Autodesk Fusion 360 part; units mm, degrees
(part 4 of 6)
  spline S27 degree 5 poles (23.2819, -10.1545) (23.2739, -10.1416) (23.2579, -10.1158) (23.2338, -10.0772) (23.2015, -10.026) (23.1609, -9.9622) (23.12, -9.8988) (23.0788, -9.8357) (23.0374, -9.7729) (22.9956, -9.7104) (22.9537, -9.6483) (22.9114, -9.5865) (22.8688, -9.525) (22.826, -9.4639) (22.7829, -9.4031) (22.7396, -9.3426) (22.6959, -9.2826) (22.652, -9.2228) (22.6078, -9.1634) (22.5634, -9.1044) (22.5186, -9.0458) (22.4736, -8.9875) (22.4284, -8.9296) (22.3828, -8.872) (22.337, -8.8148) (22.2909, -8.7581) (22.2445, -8.7017) (22.1979, -8.6456) (22.151, -8.59) (22.1038, -8.5348) (22.0563, -8.48) (22.0086, -8.4256) (21.9606, -8.3716) (21.9123, -8.318) (21.8638, -8.2649) (21.8149, -8.2122) (21.7658, -8.1599) (21.7164, -8.108) (21.6668, -8.0566) (21.6168, -8.0056) (21.5666, -7.9551) (21.5161, -7.9051) (21.4653, -7.8556) (21.4143, -7.8065) (21.3629, -7.7579) (21.3113, -7.7099) (21.2594, -7.6623) (21.2072, -7.6152) (21.1547, -7.5686) (21.1019, -7.5225) (21.0489, -7.477) (20.9955, -7.4321) (20.9418, -7.3878) (20.8878, -7.3441) (20.8335, -7.3011) (20.7788, -7.2586) (20.7239, -7.2166) (20.6688, -7.1752) (20.6133, -7.1344) (20.5575, -7.0942) (20.5014, -7.0549) (20.4448, -7.0164) (20.3878, -6.979) (20.3303, -6.9426) (20.2724, -6.907) (20.2143, -6.8722) (20.1559, -6.8378) (20.0973, -6.8039) (20.0385, -6.7707) (19.9791, -6.7389) (19.919, -6.7091) (19.8699, -6.6876) (19.8324, -6.673) (19.8071, -6.6641) (19.7944, -6.6598) knots -1 -1 -1 -1 -1 -1 -0.98571429 -0.97142857 -0.95714286 -0.94285714 -0.92857143 -0.91428571 -0.9 -0.88571429 -0.87142857 -0.85714286 -0.84285714 -0.82857143 -0.81428571 -0.8 -0.78571429 -0.77142857 -0.75714286 -0.74285714 -0.72857143 -0.71428571 -0.7 -0.68571429 -0.67142857 -0.65714286 -0.64285714 -0.62857143 -0.61428571 -0.6 -0.58571429 -0.57142857 -0.55714286 -0.54285714 -0.52857143 -0.51428571 -0.5 -0.48571429 -0.47142857 -0.45714286 -0.44285714 -0.42857143 -0.41428571 -0.4 -0.38571429 -0.37142857 -0.35714286 -0.34285714 -0.32857143 -0.31428571 -0.3 -0.28571429 -0.27142857 -0.25714286 -0.24285714 -0.22857143 -0.21428571 -0.2 -0.18571429 -0.17142857 -0.15714286 -0.14285714 -0.12857143 -0.11428571 -0.1 -0.08571429 -0.07142857 -0.05714286 -0.04285714 -0.02857143 -0.01428571 0 0 0 0 0 0
  line L27 (19.7944, -6.6598) -> (18.8495, -6.3414)
  arc A59 (17.8163, -4.4521) -> (18.8495, -6.3414) centre (19.3565, -4.837) ccw
  line L28 (3.3592, 13.8919) -> (10.16, 13.8919)
  line L29 (10.16, 13.8919) -> (10.16, 101.6)
  line L30 (10.16, 101.6) -> (3.3592, 101.6)
  line L31 (3.3592, 35.7199) -> (-12.5468, 19.2505)
  line L32 (-10.3768, 14.5152) -> (3.3592, 18.3604)
  line L33 (-12.5468, 19.2505) -> (-10.3768, 14.5152)
  line L34 (3.3592, 101.6) -> (3.3592, 35.7199)
  line L35 (3.3592, 18.3604) -> (3.3592, 13.8919)
  line L36 (-55.9735, 14.1018) -> (-55.9735, 101.81)
  line L37 (-35.4367, 14.7251) -> (-49.1726, 18.5703)
  line L38 (-55.9735, 101.81) -> (-49.1726, 101.81)
  line L39 (-49.1726, 18.5703) -> (-49.1726, 14.1018)
  line L40 (-49.1726, 101.81) -> (-49.1726, 35.9298)
  line L41 (-49.1726, 35.9298) -> (-33.2667, 19.4605)
  line L42 (-33.2667, 19.4605) -> (-35.4367, 14.7251)
  line L43 (-49.1726, 14.1018) -> (-55.9735, 14.1018)
  constraint horizontal L28
  constraint vertical L29
  constraint horizontal L30
  constraint vertical L34
  constraint coincident S10 L31.end
  constraint coincident L32.end L34
  constraint collinear L34 L35
  constraint perpendicular L36 L43
extrude "Extrude3'" add sketch "Sketch3 (3)" against normal blind 12.7 contours A15 A16 A17 L6 S6 A18 S7 L7 A19 A20 A21 L8 S8 A22 S9 L9 A23 A24 A25 L10 S10 L29 L30 L31 L34 | L36 L37 L38 L39 L40 L41 L42 L43 sketch seen with x (0.965926, -0.258819, 0) y (0.258819, 0.965926, 0) z (0, 0, 1) at (44.1308, -10.9509, 0) bodies 2 makes body 3 at (65.5892, 29.8778, 8.4667) in component "Spur Gear (14 teeth) (1)"
sketch "Sketch4" plane through (3.3592, 0, 0) normal (-1, 0, 0) x (0, 0, 1)
  line L0 (12.7, 35.7199) -> (12.7, 101.6)
  line L1 (12.7, 101.6) -> (0, 101.6)
  line L2 (0, 101.6) -> (0, 35.7199)
  line L3 (0, 35.7199) -> (12.7, 35.7199)
  line L4 (12.7, 101.6) -> (23.6482, 101.6)
  line L5 (23.6482, 101.6) -> (23.6482, 52.5233)
  line L6 (12.9467, 36.0985) -> (12.7, 36.0985)
  line L7 (12.7, 36.0985) -> (12.7, 101.6)
  line L8 (12.7, 35.7199) -> (23.6482, 52.5233)
  constraint horizontal L4
  constraint vertical L5
  constraint horizontal L6
  constraint vertical L7
  constraint coincident L0.end L1.start
  constraint coincident L0.start L3.end
  constraint coincident L8 L6.start
extrude "Extrude4" add sketch "Sketch4" against normal blind 7.62 contours L0 L4 L5 L6 L7 L8 sketch seen with x (0.965926, -0.258819, 0) y (0.258819, 0.965926, 0) z (0, 0, 1) at (44.1308, -10.9509, 0) bodies 3 in component "Spur Gear (14 teeth) (1)"
ref_plane "WorkPlane1" through (-15.6908, 68.6599, 11.8241) normal (-1, 0, 0) x (0, 1, 0)
sketch "Sketch5" plane through (-15.6908, 0, 0) normal (-1, 0, 0) x (0, 0, 1)
  point P0 (12.6888, 89.7764)
sketch "Sketch6" plane through (3.3592, 0, 0) normal (-1, 0, 0) x (0, 0, 1)
  line L0 (23.6482, 101.6) -> (0, 101.6)
  line L1 (0, 101.6) -> (0, 35.7199)
  line L2 (0, 35.7199) -> (12.7, 35.7199)
  line L3 (12.7, 35.7199) -> (12.7, 36.0985)
  line L4 (12.7, 36.0985) -> (12.9467, 36.0985)
  line L5 (12.9467, 36.0985) -> (23.6482, 52.5233)
  line L6 (23.6482, 52.5233) -> (23.6482, 101.6)
  line L7 (0, 101.6) -> (23.6482, 101.6)
  line L8 (23.6482, 101.6) -> (23.6482, 77.0617)
  line L9 (23.6482, 77.0617) -> (0, 77.0617)
  line L10 (0, 77.0617) -> (0, 101.6)
  constraint horizontal L7
  constraint vertical L8
  constraint horizontal L9
  constraint vertical L10
  constraint midpoint L6 L8.end
  constraint coincident L0.end L1.start
loft "Loft1" add profiles "Sketch6" section 1 contours L0 L1 L6 L7 L8 L9 L10 sketch seen with x (0.965926, -0.258819, 0) y (0.258819, 0.965926, 0) z (0, 0, 1) at (44.1308, -10.9509, 0) section 2 point at (52.2104, 79.8275, 12.6888) bodies 3 in component "Spur Gear (14 teeth) (1)"
sketch "Sketch7" plane through (3.3592, 0, 0) normal (-1, 0, 0) x (0, 0, 1)
  line L0 (23.6482, 77.0617) -> (0, 77.0617)
  line L1 (0, 77.0617) -> (0, 35.7199)
  line L2 (0, 35.7199) -> (12.7, 35.7199)
  line L3 (12.7, 35.7199) -> (12.7, 36.0985)
  line L4 (12.7, 36.0985) -> (12.9467, 36.0985)
  line L5 (12.9467, 36.0985) -> (23.6482, 52.5233)
  line L6 (23.6482, 52.5233) -> (23.6482, 77.0617)
  line L7 (0, 77.0617) -> (23.6482, 77.0617)
  line L8 (23.6482, 77.0617) -> (23.6482, 55.8032)
  line L9 (23.6482, 55.8032) -> (0, 55.8032)
  line L10 (0, 55.8032) -> (0, 77.0617)
  constraint horizontal L7
  constraint vertical L8
  constraint horizontal L9
  constraint vertical L10
  constraint coincident L6 L8.end
  constraint coincident L0.end L1.start
ref_plane "WorkPlane2" through (-15.6908, 66.4325, 11.8241) normal (-1, 0, 0) x (0, 0, 1)
sketch "Sketch8" plane through (-15.6908, 0, 0) normal (-1, 0, 0) x (0, 0, 1)
  point P0 (12.5523, 67.1276)
loft "Loft2" add profiles "Sketch7" section 1 contours L0 L1 L6 L7 L8 L9 L10 sketch seen with x (0.965926, -0.258819, 0) y (0.258819, 0.965926, 0) z (0, 0, 1) at (44.1308, -10.9509, 0) section 2 point at (46.3485, 57.9505, 12.5523) bodies 3 in component "Spur Gear (14 teeth) (1)"
sketch "Sketch9" plane through (-49.1726, 0, 0) normal (1, 0, 0) x (0, 0, -1)
  line L0 (-12.7, 101.81) -> (-12.7, 35.9298)
  line L1 (-12.7, 35.9298) -> (0, 35.9298)
  line L2 (0, 35.9298) -> (0, 101.81)
  line L3 (0, 101.81) -> (-12.7, 101.81)
  line L4 (0, 101.81) -> (-23.6474, 101.81)
  line L5 (-23.6474, 101.81) -> (-23.6474, 52.5287)
  line L6 (0, 35.8833) -> (0, 101.81)
  line L7 (-12.7, 35.9298) -> (-23.6474, 52.5287)
  dimension "d33" = 23.6474
  constraint horizontal L4
  constraint vertical L5
  constraint vertical L6
  constraint coincident L2.end L3.start
  constraint coincident L0.end L1.start
  measures "d33" distance of L2.end L4.end
extrude "Extrude5" add sketch "Sketch9" against normal blind 6.731 contours L0 L4 L5 L7 sketch seen with x (0.965926, -0.258819, 0) y (0.258819, 0.965926, 0) z (0, 0, 1) at (44.1308, -10.9509, 0) bodies 2 in component "Spur Gear (14 teeth) (1)"
sketch "Sketch10" plane through (-49.1726, 0, 0) normal (1, 0, 0) x (0, 0, -1)
  line L0 (-12.7, 35.9298) -> (0, 35.9298)
  line L1 (0, 35.9298) -> (0, 101.81)
  line L2 (0, 101.81) -> (-23.6474, 101.81)
  line L3 (-23.6474, 101.81) -> (-23.6474, 52.5287)
  line L4 (-23.6474, 52.5287) -> (-12.7, 35.9298)
  line L5 (-23.6474, 101.81) -> (-0.1184, 101.81)
  line L6 (-0.1184, 101.81) -> (-0.1184, 77.2736)
  line L7 (-0.1184, 77.2736) -> (-23.6474, 77.2736)
  line L8 (-23.6474, 77.2736) -> (-23.6474, 101.81)
  line L9 (-23.6474, 77.2736) -> (0, 77.2736)
  line L10 (0, 77.2736) -> (0, 52.4632)
  line L11 (0, 52.4632) -> (-23.6474, 52.4632)
  line L12 (-23.6474, 52.4632) -> (-23.6474, 77.2736)
  dimension "d36" = 24.5364
  constraint horizontal L5
  constraint vertical L6
  constraint horizontal L7
  constraint vertical L8
  constraint coincident L2.end L3.start
  constraint horizontal L9
  constraint vertical L10
  constraint horizontal L11
  constraint vertical L12
  constraint coincident L1 L10.end
  measures "d36" distance of L2.end L7.end
ref_plane "WorkPlane3" through (-30.1226, 89.5418, 11.8829) normal (1, 0, 0) x (0, 0, -1)
ref_plane "WorkPlane4" through (-30.1226, 64.8684, 11.8237) normal (1, 0, 0) x (0, 0, -1)
sketch "Sketch11" plane through (-30.1226, 0, 0) normal (1, 0, 0) x (0, 0, -1)
  point P0 (-11.0515, 90.4417)
sketch "Sketch12" plane through (-49.1726, 0, 0) normal (1, 0, 0) x (0, 0, -1)
sketch "Sketch13" plane through (-30.1226, 0, 0) normal (1, 0, 0) x (0, 0, -1)
  point P0 (-11.1758, 64.0599)
loft "Loft3" add profiles "Sketch10" section 1 contours L2 L3 L5 L6 L7 L8 L9 sketch seen with x (0.965926, -0.258819, 0) y (0.258819, 0.965926, 0) z (0, 0, 1) at (44.1308, -10.9509, 0) section 2 point at (38.4426, 84.2054, 11.0515) bodies 2 in component "Spur Gear (14 teeth) (1)"
sketch "Sketch14" plane through (-49.1726, 0, 0) normal (1, 0, 0) x (0, 0, -1)
  line L0 (-0.1184, 101.81) -> (-0.1184, 77.2736)
  line L1 (-0.1184, 77.2736) -> (-23.6474, 77.2736)
  line L2 (-23.6474, 77.2736) -> (-23.6474, 52.5287)
  line L3 (-23.6474, 52.5287) -> (-12.7, 35.9298)
  line L4 (-12.7, 35.9298) -> (0, 35.9298)
  line L5 (0, 35.9298) -> (0, 101.81)
  line L6 (0, 101.81) -> (-0.1184, 101.81)
  line L7 (-23.6474, 77.2736) -> (0, 77.2736)
  line L8 (0, 77.2736) -> (0, 52.6508)
  line L9 (0, 52.6508) -> (-23.6474, 52.6508)
  line L10 (-23.6474, 52.6508) -> (-23.6474, 77.2736)
  constraint horizontal L7
  constraint vertical L8
  constraint horizontal L9
  constraint vertical L10
  constraint coincident L5 L8.end
  constraint coincident L1.end L2.start
loft "Loft4" add profiles "Sketch14" section 1 contours L1 L2 L5 L7 L8 L9 L10 sketch seen with x (0.965926, -0.258819, 0) y (0.258819, 0.965926, 0) z (0, 0, 1) at (44.1308, -10.9509, 0) section 2 point at (31.6145, 58.7226, 11.1758) bodies 2 in component "Spur Gear (14 teeth) (1)"
sketch "Sketch15" plane through (0, 0, 12.7) normal (0, 0, 1) x (1, 0, 0)
  line L0 (-55.9036, 35.9298) -> (-55.9036, 101.81)
  line L1 (-55.9036, 101.81) -> (-55.9735, 101.81)
  line L2 (-55.9735, 101.81) -> (-55.9735, 21.7403)
  spline S0 degree 5 poles (-55.9735, 21.7403) (-55.9837, 21.7467) (-56.0067, 21.761) (-56.0426, 21.7832) (-56.0913, 21.8132) (-56.1531, 21.8508) (-56.2177, 21.8896) (-56.2826, 21.928) (-56.3479, 21.9663) (-56.4003, 21.9966) (-56.4398, 22.0192) (-56.4661, 22.0343) (-56.4794, 22.0418) knots 0.888467 0.888467 0.888467 0.888467 0.888467 0.888467 0.9 0.914286 0.928571 0.942857 0.957143 0.971429 0.985714 1 1 1 1 1 1
  arc A0 (-56.4794, 22.0418) -> (-58.1639, 21.1514) centre (-45.4614, -0.8441) ccw
  spline S1 degree 5 poles (-58.1639, 21.1514) (-58.1652, 21.1363) (-58.1676, 21.106) (-58.1712, 21.0607) (-58.1756, 21.0003) (-58.1808, 20.9248) (-58.1856, 20.8495) (-58.1899, 20.7743) (-58.1939, 20.6991) (-58.1974, 20.6241) (-58.2005, 20.5492) (-58.2032, 20.4743) (-58.2055, 20.3996) (-58.2073, 20.325) (-58.2087, 20.2505) (-58.2097, 20.1761) (-58.2103, 20.1019) (-58.2104, 20.0277) (-58.2101, 19.9537) (-58.2094, 19.8798) (-58.2083, 19.8061) (-58.2067, 19.7325) (-58.2046, 19.659) (-58.2022, 19.5856) (-58.1992, 19.5124) (-58.1959, 19.4394) (-58.1921, 19.3665) (-58.1878, 19.2937) (-58.1831, 19.2211) (-58.1779, 19.1486) (-58.1723, 19.0763) (-58.1662, 19.0042) (-58.1596, 18.9323) (-58.1526, 18.8605) (-58.1451, 18.7889) (-58.1371, 18.7175) (-58.1286, 18.6463) (-58.1197, 18.5752) (-58.1102, 18.5044) (-58.1003, 18.4337) (-58.0899, 18.3632) (-58.079, 18.293) (-58.0675, 18.223) (-58.0556, 18.1532) (-58.0431, 18.0836) (-58.0301, 18.0143) (-58.0166, 17.9451) (-58.0026, 17.8763) (-57.988, 17.8076) (-57.9729, 17.7392) (-57.9572, 17.6711) (-57.941, 17.6033) (-57.9241, 17.5357) (-57.9065, 17.4685) (-57.8884, 17.4016) (-57.8697, 17.335) (-57.8504, 17.2686) (-57.8306, 17.2025) (-57.8103, 17.1368) (-57.7892, 17.0713) (-57.7674, 17.0063) (-57.7447, 16.9418) (-57.7211, 16.8778) (-57.6965, 16.8144) (-57.671, 16.7514) (-57.6449, 16.6888) (-57.6183, 16.6265) (-57.5913, 16.5645) (-57.5637, 16.5029) (-57.5349, 16.442) (-57.5041, 16.3822) (-57.4774, 16.3358) (-57.4559, 16.3018) (-57.4408, 16.2796) (-57.4332, 16.2686) knots -1 -1 -1 -1 -1 -1 -0.98571429 -0.97142857 -0.95714286 -0.94285714 -0.92857143 -0.91428571 -0.9 -0.88571429 -0.87142857 -0.85714286 -0.84285714 -0.82857143 -0.81428571 -0.8 -0.78571429 -0.77142857 -0.75714286 -0.74285714 -0.72857143 -0.71428571 -0.7 -0.68571429 -0.67142857 -0.65714286 -0.64285714 -0.62857143 -0.61428571 -0.6 -0.58571429 -0.57142857 -0.55714286 -0.54285714 -0.52857143 -0.51428571 -0.5 -0.48571429 -0.47142857 -0.45714286 -0.44285714 -0.42857143 -0.41428571 -0.4 -0.38571429 -0.37142857 -0.35714286 -0.34285714 -0.32857143 -0.31428571 -0.3 -0.28571429 -0.27142857 -0.25714286 -0.24285714 -0.22857143 -0.21428571 -0.2 -0.18571429 -0.17142857 -0.15714286 -0.14285714 -0.12857143 -0.11428571 -0.1 -0.08571429 -0.07142857 -0.05714286 -0.04285714 -0.02857143 -0.01428571 0 0 0 0 0 0
  line L3 (-57.4332, 16.2686) -> (-56.862, 15.4514)
  arc A1 (-57.1526, 13.3178) -> (-56.862, 15.4514) centre (-58.1632, 14.542) ccw
  arc A2 (-57.1526, 13.3178) -> (-57.7226, 12.8272) centre (-45.4614, -0.8441) ccw
  arc A3 (-59.8757, 12.8579) -> (-57.7226, 12.8272) centre (-58.7825, 14.009) ccw
  line L4 (-59.8757, 12.8579) -> (-60.5987, 13.5444)
  spline S2 degree 5 poles (-60.5987, 13.5444) (-60.6084, 13.5537) (-60.6281, 13.5719) (-60.6585, 13.5982) (-60.7005, 13.6316) (-60.7549, 13.6709) (-60.8109, 13.7084) (-60.8677, 13.745) (-60.925, 13.7809) (-60.9826, 13.8165) (-61.0407, 13.8516) (-61.0991, 13.8862) (-61.1582, 13.92) (-61.2179, 13.9529) (-61.2783, 13.9849) (-61.3394, 14.0162) (-61.401, 14.0467) (-61.463, 14.0767) (-61.5253, 14.1061) (-61.5881, 14.135) (-61.6512, 14.1635) (-61.7146, 14.1914) (-61.7785, 14.2187) (-61.8428, 14.2455) (-61.9074, 14.2717) (-61.9724, 14.2973) (-62.0378, 14.3225) (-62.1035, 14.3471) (-62.1695, 14.3712) (-62.2359, 14.3949) (-62.3025, 14.4181) (-62.3695, 14.4408) (-62.4367, 14.463) (-62.5042, 14.4848) (-62.5721, 14.506) (-62.6402, 14.5268) (-62.7086, 14.5472) (-62.7772, 14.5671) (-62.8461, 14.5865) (-62.9153, 14.6055) (-62.9847, 14.624) (-63.0544, 14.6421) (-63.1243, 14.6598) (-63.1945, 14.677) (-63.2649, 14.6938) (-63.3356, 14.7101) (-63.4064, 14.726) (-63.4775, 14.7415) (-63.5488, 14.7566) (-63.6204, 14.7712) (-63.6921, 14.7854) (-63.7641, 14.7992) (-63.8362, 14.8126) (-63.9086, 14.8256) (-63.9811, 14.8381) (-64.0539, 14.8503) (-64.1269, 14.862) (-64.2, 14.8733) (-64.2733, 14.8842) (-64.3468, 14.8947) (-64.4205, 14.9048) (-64.4944, 14.9145) (-64.5685, 14.9238) (-64.6427, 14.9327) (-64.7171, 14.9412) (-64.7916, 14.9493) (-64.8664, 14.957) (-64.9412, 14.9643) (-65.0163, 14.9712) (-65.0915, 14.9777) (-65.1668, 14.9838) (-65.2272, 14.9884) (-65.2726, 14.9917) (-65.3029, 14.9938) (-65.318, 14.9948) knots 0 0 0 0 0 0 0.01428571 0.02857143 0.04285714 0.05714286 0.07142857 0.08571429 0.1 0.11428571 0.12857143 0.14285714 0.15714286 0.17142857 0.18571429 0.2 0.21428571 0.22857143 0.24285714 0.25714286 0.27142857 0.28571429 0.3 0.31428571 0.32857143 0.34285714 0.35714286 0.37142857 0.38571429 0.4 0.41428571 0.42857143 0.44285714 0.45714286 0.47142857 0.48571429 0.5 0.51428571 0.52857143 0.54285714 0.55714286 0.57142857 0.58571429 0.6 0.61428571 0.62857143 0.64285714 0.65714286 0.67142857 0.68571429 0.7 0.71428571 0.72857143 0.74285714 0.75714286 0.77142857 0.78571429 0.8 0.81428571 0.82857143 0.84285714 0.85714286 0.87142857 0.88571429 0.9 0.91428571 0.92857143 0.94285714 0.95714286 0.97142857 0.98571429 1 1 1 1 1 1
  arc A4 (-65.318, 14.9948) -> (-66.4495, 13.4617) centre (-45.4614, -0.8441) ccw
  spline S3 degree 5 poles (-66.4495, 13.4617) (-66.4441, 13.4476) (-66.4331, 13.4192) (-66.4166, 13.3768) (-66.3945, 13.3205) (-66.3664, 13.2503) (-66.338, 13.1803) (-66.3093, 13.1107) (-66.2802, 13.0413) (-66.2509, 12.9721) (-66.2211, 12.9033) (-66.1911, 12.8347) (-66.1607, 12.7664) (-66.13, 12.6984) (-66.099, 12.6306) (-66.0676, 12.5632) (-66.0359, 12.496) (-66.0039, 12.4292) (-65.9715, 12.3626) (-65.9388, 12.2964) (-65.9057, 12.2304) (-65.8723, 12.1648) (-65.8386, 12.0994) (-65.8046, 12.0344) (-65.7702, 11.9697) (-65.7354, 11.9054) (-65.7004, 11.8413) (-65.665, 11.7776) (-65.6292, 11.7143) (-65.5931, 11.6512) (-65.5567, 11.5885) (-65.5199, 11.5262) (-65.4828, 11.4642) (-65.4453, 11.4026) (-65.4074, 11.3414) (-65.3693, 11.2805) (-65.3307, 11.22) (-65.2918, 11.1599) (-65.2526, 11.1001) (-65.213, 11.0408) (-65.1731, 10.9818) (-65.1327, 10.9233) (-65.0921, 10.8651) (-65.051, 10.8074) (-65.0096, 10.7502) (-64.9678, 10.6933) (-64.9256, 10.6369) (-64.8831, 10.5809) (-64.8402, 10.5254) (-64.7969, 10.4703) (-64.7532, 10.4158) (-64.7091, 10.3617) (-64.6646, 10.3082) (-64.6196, 10.2552) (-64.5743, 10.2028) (-64.5285, 10.1509) (-64.4824, 10.0995) (-64.4359, 10.0485) (-64.389, 9.9981) (-64.3416, 9.9483) (-64.2938, 9.8992) (-64.2453, 9.8509) (-64.1963, 9.8035) (-64.1466, 9.757) (-64.0963, 9.7113) (-64.0456, 9.6663) (-63.9947, 9.6217) (-63.9434, 9.5775) (-63.8918, 9.534) (-63.8394, 9.4916) (-63.7858, 9.4511) (-63.7415, 9.4209) (-63.7074, 9.3996) (-63.6842, 9.3861) (-63.6725, 9.3795) knots -1 -1 -1 -1 -1 -1 -0.98571429 -0.97142857 -0.95714286 -0.94285714 -0.92857143 -0.91428571 -0.9 -0.88571429 -0.87142857 -0.85714286 -0.84285714 -0.82857143 -0.81428571 -0.8 -0.78571429 -0.77142857 -0.75714286 -0.74285714 -0.72857143 -0.71428571 -0.7 -0.68571429 -0.67142857 -0.65714286 -0.64285714 -0.62857143 -0.61428571 -0.6 -0.58571429 -0.57142857 -0.55714286 -0.54285714 -0.52857143 -0.51428571 -0.5 -0.48571429 -0.47142857 -0.45714286 -0.44285714 -0.42857143 -0.41428571 -0.4 -0.38571429 -0.37142857 -0.35714286 -0.34285714 -0.32857143 -0.31428571 -0.3 -0.28571429 -0.27142857 -0.25714286 -0.24285714 -0.22857143 -0.21428571 -0.2 -0.18571429 -0.17142857 -0.15714286 -0.14285714 -0.12857143 -0.11428571 -0.1 -0.08571429 -0.07142857 -0.05714286 -0.04285714 -0.02857143 -0.01428571 0 0 0 0 0 0
  line L5 (-63.6725, 9.3795) -> (-62.8034, 8.891)
  arc A5 (-62.1394, 6.8427) -> (-62.8034, 8.891) centre (-63.5812, 7.5071) ccw
  arc A6 (-62.1394, 6.8427) -> (-62.4401, 6.1534) centre (-45.4614, -0.8441) ccw
  arc A7 (-64.3933, 5.2468) -> (-62.4401, 6.1534) centre (-63.9079, 6.7583) ccw
  line L6 (-64.3933, 5.2468) -> (-65.3426, 5.5517)
  spline S4 degree 5 poles (-65.3426, 5.5517) (-65.3554, 5.5558) (-65.381, 5.5636) (-65.4198, 5.5742) (-65.4721, 5.586) (-65.5382, 5.5978) (-65.6049, 5.6074) (-65.672, 5.6156) (-65.7392, 5.6232) (-65.8066, 5.6302) (-65.8741, 5.6367) (-65.9417, 5.6424) (-66.0096, 5.6473) (-66.0777, 5.651) (-66.1461, 5.6537) (-66.2146, 5.6553) (-66.2833, 5.6561) (-66.3522, 5.6562) (-66.4212, 5.6557) (-66.4903, 5.6545) (-66.5594, 5.6528) (-66.6287, 5.6504) (-66.6981, 5.6473) (-66.7676, 5.6435) (-66.8373, 5.6391) (-66.907, 5.634) (-66.9768, 5.6283) (-67.0467, 5.6219) (-67.1166, 5.615) (-67.1867, 5.6076) (-67.2568, 5.5996) (-67.3269, 5.591) (-67.3971, 5.5818) (-67.4674, 5.5721) (-67.5378, 5.5619) (-67.6082, 5.551) (-67.6786, 5.5397) (-67.7491, 5.5278) (-67.8196, 5.5154) (-67.8902, 5.5025) (-67.9608, 5.4891) (-68.0314, 5.4752) (-68.1021, 5.4607) (-68.1727, 5.4458) (-68.2435, 5.4304) (-68.3142, 5.4145) (-68.3849, 5.398) (-68.4557, 5.3811) (-68.5265, 5.3638) (-68.5973, 5.3459) (-68.6681, 5.3276) (-68.7389, 5.3088) (-68.8097, 5.2896) (-68.8806, 5.2699) (-68.9514, 5.2497) (-69.0222, 5.229) (-69.093, 5.208) (-69.1638, 5.1864) (-69.2346, 5.1644) (-69.3054, 5.142) (-69.3762, 5.1191) (-69.447, 5.0958) (-69.5177, 5.072) (-69.5885, 5.0479) (-69.6592, 5.0232) (-69.7299, 4.9982) (-69.8005, 4.9727) (-69.8712, 4.9468) (-69.9418, 4.9204) (-70.0123, 4.8937) (-70.0829, 4.8665) (-70.1393, 4.8444) (-70.1816, 4.8277) (-70.2098, 4.8164) (-70.2239, 4.8108) knots 0 0 0 0 0 0 0.01428571 0.02857143 0.04285714 0.05714286 0.07142857 0.08571429 0.1 0.11428571 0.12857143 0.14285714 0.15714286 0.17142857 0.18571429 0.2 0.21428571 0.22857143 0.24285714 0.25714286 0.27142857 0.28571429 0.3 0.31428571 0.32857143 0.34285714 0.35714286 0.37142857 0.38571429 0.4 0.41428571 0.42857143 0.44285714 0.45714286 0.47142857 0.48571429 0.5 0.51428571 0.52857143 0.54285714 0.55714286 0.57142857 0.58571429 0.6 0.61428571 0.62857143 0.64285714 0.65714286 0.67142857 0.68571429 0.7 0.71428571 0.72857143 0.74285714 0.75714286 0.77142857 0.78571429 0.8 0.81428571 0.82857143 0.84285714 0.85714286 0.87142857 0.88571429 0.9 0.91428571 0.92857143 0.94285714 0.95714286 0.97142857 0.98571429 1 1 1 1 1 1
  arc A8 (-70.2239, 4.8108) -> (-70.5781, 2.9386) centre (-45.4614, -0.8441) ccw
  spline S5 degree 5 poles (-70.5781, 2.9386) (-70.5671, 2.9282) (-70.5449, 2.9074) (-70.5117, 2.8764) (-70.4672, 2.8352) (-70.4115, 2.7841) (-70.3556, 2.7334) (-70.2995, 2.6831) (-70.2432, 2.6332) (-70.1867, 2.5837) (-70.1301, 2.5345) (-70.0732, 2.4858) (-70.0162, 2.4374) (-69.959, 2.3894) (-69.9017, 2.3419) (-69.8442, 2.2947) (-69.7865, 2.248) (-69.7286, 2.2016) (-69.6705, 2.1557) (-69.6123, 2.1102) (-69.5539, 2.0651) (-69.4954, 2.0205) (-69.4367, 1.9763) (-69.3778, 1.9325) (-69.3187, 1.8891) (-69.2595, 1.8462) (-69.2001, 1.8037) (-69.1406, 1.7617) (-69.0809, 1.7201) (-69.021, 1.679) (-68.961, 1.6383) (-68.9008, 1.5981) (-68.8404, 1.5584) (-68.7799, 1.5191) (-68.7193, 1.4804) (-68.6584, 1.4421) (-68.5975, 1.4043) (-68.5364, 1.367) (-68.4751, 1.3302) (-68.4137, 1.2939) (-68.3521, 1.2581) (-68.2903, 1.2228) (-68.2285, 1.1881) (-68.1664, 1.1539) (-68.1043, 1.1203) (-68.0419, 1.0873) (-67.9795, 1.0547) (-67.9169, 1.0227) (-67.8541, 0.9913) (-67.7912, 0.9605) (-67.7282, 0.9303) (-67.665, 0.9007) (-67.6017, 0.8718) (-67.5382, 0.8436) (-67.4746, 0.816) (-67.4108, 0.7891) (-67.347, 0.7628) (-67.2829, 0.7371) (-67.2188, 0.712) (-67.1546, 0.6877) (-67.0901, 0.6642) (-67.0255, 0.6417) (-66.9608, 0.6203) (-66.8958, 0.6) (-66.8307, 0.5806) (-66.7655, 0.562) (-66.7002, 0.5439) (-66.6349, 0.5264) (-66.5695, 0.5096) (-66.5039, 0.4941) (-66.438, 0.4809) (-66.3851, 0.4729) (-66.3451, 0.4685) (-66.3183, 0.4664) (-66.3049, 0.4656) knots -1 -1 -1 -1 -1 -1 -0.98571429 -0.97142857 -0.95714286 -0.94285714 -0.92857143 -0.91428571 -0.9 -0.88571429 -0.87142857 -0.85714286 -0.84285714 -0.82857143 -0.81428571 -0.8 -0.78571429 -0.77142857 -0.75714286 -0.74285714 -0.72857143 -0.71428571 -0.7 -0.68571429 -0.67142857 -0.65714286 -0.64285714 -0.62857143 -0.61428571 -0.6 -0.58571429 -0.57142857 -0.55714286 -0.54285714 -0.52857143 -0.51428571 -0.5 -0.48571429 -0.47142857 -0.45714286 -0.44285714 -0.42857143 -0.41428571 -0.4 -0.38571429 -0.37142857 -0.35714286 -0.34285714 -0.32857143 -0.31428571 -0.3 -0.28571429 -0.27142857 -0.25714286 -0.24285714 -0.22857143 -0.21428571 -0.2 -0.18571429 -0.17142857 -0.15714286 -0.14285714 -0.12857143 -0.11428571 -0.1 -0.08571429 -0.07142857 -0.05714286 -0.04285714 -0.02857143 -0.01428571 0 0 0 0 0 0
  line L7 (-66.3049, 0.4656) -> (-65.3099, 0.4026)
  arc A9 (-63.8229, -1.1549) -> (-65.3099, 0.4026) centre (-65.4102, -1.1818) ccw
  arc A10 (-63.8229, -1.1549) -> (-63.7948, -1.9064) centre (-45.4614, -0.8441) ccw
  arc A11 (-65.1612, -3.5706) -> (-63.7948, -1.9064) centre (-65.3797, -1.9982) ccw
  line L8 (-65.1612, -3.5706) -> (-66.1488, -3.7078)
  spline S6 degree 5 poles (-66.1488, -3.7078) (-66.1621, -3.7097) (-66.1886, -3.7138) (-66.2281, -3.7211) (-66.2804, -3.7331) (-66.3451, -3.7512) (-66.4093, -3.7715) (-66.4733, -3.7931) (-66.5371, -3.8155) (-66.6009, -3.8384) (-66.6645, -3.8619) (-66.728, -3.886) (-66.7912, -3.9111) (-66.8542, -3.9373) (-66.9169, -3.9646) (-66.9794, -3.9928) (-67.0417, -4.0219) (-67.1038, -4.0517) (-67.1657, -4.0821) (-67.2274, -4.1131) (-67.289, -4.1447) (-67.3504, -4.177) (-67.4116, -4.2098) (-67.4725, -4.2434) (-67.5333, -4.2776) (-67.5939, -4.3124) (-67.6544, -4.3479) (-67.7146, -4.3839) (-67.7746, -4.4205) (-67.8345, -4.4576) (-67.8942, -4.4952) (-67.9536, -4.5334) (-68.0129, -4.5721) (-68.072, -4.6114) (-68.131, -4.6511) (-68.1897, -4.6914) (-68.2482, -4.7322) (-68.3066, -4.7735) (-68.3648, -4.8152) (-68.4227, -4.8575) (-68.4805, -4.9002) (-68.5381, -4.9434) (-68.5955, -4.9871) (-68.6527, -5.0312) (-68.7097, -5.0758) (-68.7666, -5.1208) (-68.8232, -5.1663) (-68.8796, -5.2122) (-68.9359, -5.2586) (-68.9919, -5.3054) (-69.0477, -5.3526) (-69.1034, -5.4003) (-69.1588, -5.4483) (-69.2141, -5.4968) (-69.2692, -5.5457) (-69.324, -5.5951) (-69.3787, -5.6448) (-69.4331, -5.6949) (-69.4874, -5.7454) (-69.5414, -5.7964) (-69.5953, -5.8477) (-69.6489, -5.8994) (-69.7023, -5.9515) (-69.7556, -6.004) (-69.8086, -6.0569) (-69.8614, -6.1101) (-69.914, -6.1637) (-69.9664, -6.2177) (-70.0186, -6.2721) (-70.0706, -6.3268) (-70.1223, -6.3819) (-70.1636, -6.4263) (-70.1944, -6.4597) (-70.215, -6.4821) (-70.2252, -6.4933) knots 0 0 0 0 0 0 0.01428571 0.02857143 0.04285714 0.05714286 0.07142857 0.08571429 0.1 0.11428571 0.12857143 0.14285714 0.15714286 0.17142857 0.18571429 0.2 0.21428571 0.22857143 0.24285714 0.25714286 0.27142857 0.28571429 0.3 0.31428571 0.32857143 0.34285714 0.35714286 0.37142857 0.38571429 0.4 0.41428571 0.42857143 0.44285714 0.45714286 0.47142857 0.48571429 0.5 0.51428571 0.52857143 0.54285714 0.55714286 0.57142857 0.58571429 0.6 0.61428571 0.62857143 0.64285714 0.65714286 0.67142857 0.68571429 0.7 0.71428571 0.72857143 0.74285714 0.75714286 0.77142857 0.78571429 0.8 0.81428571 0.82857143 0.84285714 0.85714286 0.87142857 0.88571429 0.9 0.91428571 0.92857143 0.94285714 0.95714286 0.97142857 0.98571429 1 1 1 1 1 1
  arc A12 (-70.2252, -6.4933) -> (-69.7321, -8.3338) centre (-45.4614, -0.8441) ccw
  spline S7 degree 5 poles (-69.7321, -8.3338) (-69.7176, -8.3383) (-69.6886, -8.3474) (-69.6452, -8.361) (-69.5873, -8.3788) (-69.5149, -8.4006) (-69.4425, -8.422) (-69.3701, -8.443) (-69.2978, -8.4636) (-69.2254, -8.4837) (-69.153, -8.5034) (-69.0807, -8.5227) (-69.0083, -8.5415) (-68.936, -8.5599) (-68.8637, -8.5779) (-68.7914, -8.5954) (-68.7191, -8.6125) (-68.6469, -8.6291) (-68.5747, -8.6453) (-68.5025, -8.6611) (-68.4303, -8.6763) (-68.3582, -8.6912) (-68.2861, -8.7055) (-68.214, -8.7194) (-68.142, -8.7329) (-68.07, -8.7459) (-67.9981, -8.7584) (-67.9262, -8.7704) (-67.8544, -8.782) (-67.7826, -8.793) (-67.7109, -8.8036) (-67.6392, -8.8137) (-67.5676, -8.8233) (-67.496, -8.8324) (-67.4246, -8.8411) (-67.3532, -8.8492) (-67.2818, -8.8568) (-67.2106, -8.8639) (-67.1394, -8.8704) (-67.0683, -8.8765) (-66.9973, -8.882) (-66.9264, -8.887) (-66.8556, -8.8914) (-66.7849, -8.8953) (-66.7143, -8.8986) (-66.6438, -8.9014) (-66.5734, -8.9036) (-66.5031, -8.9052) (-66.4329, -8.9063) (-66.3629, -8.9068) (-66.293, -8.9067) (-66.2232, -8.9059) (-66.1536, -8.9045) (-66.0842, -8.9023) (-66.0149, -8.8995) (-65.9458, -8.8961) (-65.8768, -8.8921) (-65.808, -8.8875) (-65.7394, -8.8823) (-65.6709, -8.8763) (-65.6026, -8.8696) (-65.5347, -8.8618) (-65.467, -8.853) (-65.3997, -8.8431) (-65.3327, -8.8323) (-65.2658, -8.8208) (-65.1992, -8.8087) (-65.1327, -8.7962) (-65.0665, -8.783) (-65.0007, -8.7684) (-64.9356, -8.7517) (-64.8844, -8.736) (-64.8465, -8.7226) (-64.8215, -8.7129) (-64.809, -8.7078) knots -1 -1 -1 -1 -1 -1 -0.98571429 -0.97142857 -0.95714286 -0.94285714 -0.92857143 -0.91428571 -0.9 -0.88571429 -0.87142857 -0.85714286 -0.84285714 -0.82857143 -0.81428571 -0.8 -0.78571429 -0.77142857 -0.75714286 -0.74285714 -0.72857143 -0.71428571 -0.7 -0.68571429 -0.67142857 -0.65714286 -0.64285714 -0.62857143 -0.61428571 -0.6 -0.58571429 -0.57142857 -0.55714286 -0.54285714 -0.52857143 -0.51428571 -0.5 -0.48571429 -0.47142857 -0.45714286 -0.44285714 -0.42857143 -0.41428571 -0.4 -0.38571429 -0.37142857 -0.35714286 -0.34285714 -0.32857143 -0.31428571 -0.3 -0.28571429 -0.27142857 -0.25714286 -0.24285714 -0.22857143 -0.21428571 -0.2 -0.18571429 -0.17142857 -0.15714286 -0.14285714 -0.12857143 -0.11428571 -0.1 -0.08571429 -0.07142857 -0.05714286 -0.04285714 -0.02857143 -0.01428571 0 0 0 0 0 0
  line L9 (-64.809, -8.7078) -> (-63.8852, -8.3329)
  arc A13 (-61.8697, -9.0909) -> (-63.8852, -8.3329) centre (-63.2882, -9.8038) ccw
  arc A14 (-61.8697, -9.0909) -> (-61.5183, -9.7558) centre (-45.4614, -0.8441) ccw
  arc A15 (-62.0273, -11.8481) -> (-61.5183, -9.7558) centre (-62.9064, -10.5262) ccw
  line L10 (-62.0273, -11.8481) -> (-62.8576, -12.4002)
  spline S8 degree 5 poles (-62.8576, -12.4002) (-62.8688, -12.4076) (-62.8909, -12.4228) (-62.9233, -12.4465) (-62.9652, -12.48) (-63.0156, -12.5244) (-63.0647, -12.5705) (-63.1129, -12.6178) (-63.1607, -12.6657) (-63.2082, -12.714) (-63.2554, -12.7627) (-63.3021, -12.812) (-63.3482, -12.8621) (-63.3936, -12.913) (-63.4383, -12.9648) (-63.4823, -13.0173) (-63.5258, -13.0706) (-63.5688, -13.1243) (-63.6114, -13.1786) (-63.6535, -13.2333) (-63.6953, -13.2885) (-63.7366, -13.3442) (-63.7775, -13.4004) (-63.8179, -13.4571) (-63.8578, -13.5143) (-63.8973, -13.5719) (-63.9363, -13.6301) (-63.975, -13.6887) (-64.0132, -13.7477) (-64.051, -13.8071) (-64.0885, -13.8669) (-64.1255, -13.9271) (-64.1621, -13.9877) (-64.1984, -14.0487) (-64.2342, -14.1101) (-64.2696, -14.1719) (-64.3047, -14.234) (-64.3393, -14.2965) (-64.3736, -14.3594) (-64.4075, -14.4226) (-64.441, -14.4862) (-64.4742, -14.5501) (-64.507, -14.6143) (-64.5394, -14.6789) (-64.5714, -14.7438) (-64.603, -14.809) (-64.6343, -14.8746) (-64.6652, -14.9404) (-64.6958, -15.0066) (-64.726, -15.0731) (-64.7558, -15.1399) (-64.7853, -15.207) (-64.8144, -15.2743) (-64.8431, -15.342) (-64.8715, -15.4099) (-64.8995, -15.4782) (-64.9272, -15.5467) (-64.9545, -15.6155) (-64.9815, -15.6845) (-65.0081, -15.7539) (-65.0343, -15.8235) (-65.0602, -15.8933) (-65.0857, -15.9635) (-65.1109, -16.0339) (-65.1357, -16.1045) (-65.1602, -16.1754) (-65.1844, -16.2465) (-65.2081, -16.3179) (-65.2316, -16.3895) (-65.2547, -16.4614) (-65.2774, -16.5335) (-65.2953, -16.5914) (-65.3086, -16.6349) (-65.3174, -16.6639) (-65.3217, -16.6785) knots 0 0 0 0 0 0 0.01428571 0.02857143 0.04285714 0.05714286 0.07142857 0.08571429 0.1 0.11428571 0.12857143 0.14285714 0.15714286 0.17142857 0.18571429 0.2 0.21428571 0.22857143 0.24285714 0.25714286 0.27142857 0.28571429 0.3 0.31428571 0.32857143 0.34285714 0.35714286 0.37142857 0.38571429 0.4 0.41428571 0.42857143 0.44285714 0.45714286 0.47142857 0.48571429 0.5 0.51428571 0.52857143 0.54285714 0.55714286 0.57142857 0.58571429 0.6 0.61428571 0.62857143 0.64285714 0.65714286 0.67142857 0.68571429 0.7 0.71428571 0.72857143 0.74285714 0.75714286 0.77142857 0.78571429 0.8 0.81428571 0.82857143 0.84285714 0.85714286 0.87142857 0.88571429 0.9 0.91428571 0.92857143 0.94285714 0.95714286 0.97142857 0.98571429 1 1 1 1 1 1
  arc A16 (-65.3217, -16.6785) -> (-64.0789, -18.1227) centre (-45.4614, -0.8441) ccw
  spline S9 degree 5 poles (-64.0789, -18.1227) (-64.0638, -18.1205) (-64.0338, -18.1162) (-63.9888, -18.1095) (-63.9289, -18.1005) (-63.8542, -18.0887) (-63.7797, -18.0766) (-63.7054, -18.0641) (-63.6313, -18.0512) (-63.5573, -18.038) (-63.4836, -18.0243) (-63.41, -18.0103) (-63.3367, -17.9959) (-63.2635, -17.9811) (-63.1906, -17.9659) (-63.1179, -17.9503) (-63.0453, -17.9344) (-62.973, -17.918) (-62.9009, -17.9012) (-62.8291, -17.8841) (-62.7574, -17.8666) (-62.686, -17.8486) (-62.6148, -17.8303) (-62.5438, -17.8115) (-62.4731, -17.7924) (-62.4026, -17.7729) (-62.3324, -17.7529) (-62.2624, -17.7326) (-62.1927, -17.7118) (-62.1232, -17.6907) (-62.054, -17.6691) (-61.985, -17.6471) (-61.9163, -17.6247) (-61.8479, -17.6018) (-61.7798, -17.5786) (-61.7119, -17.5549) (-61.6444, -17.5308) (-61.5771, -17.5063) (-61.5101, -17.4813) (-61.4435, -17.4559) (-61.3771, -17.4301) (-61.311, -17.4038) (-61.2453, -17.3771) (-61.1799, -17.3499) (-61.1149, -17.3222) (-61.0502, -17.2941) (-60.9858, -17.2656) (-60.9217, -17.2366) (-60.8581, -17.2071) (-60.7947, -17.1772) (-60.7318, -17.1467) (-60.6693, -17.1158) (-60.6072, -17.0843) (-60.5456, -17.0522) (-60.4844, -17.0197) (-60.4236, -16.9866) (-60.3632, -16.9531) (-60.3032, -16.919) (-60.2436, -16.8845) (-60.1845, -16.8495) (-60.1259, -16.8138) (-60.0681, -16.7773) (-60.011, -16.74) (-59.9546, -16.7019) (-59.8989, -16.663) (-59.8437, -16.6237) (-59.7888, -16.5839) (-59.7344, -16.5438) (-59.6804, -16.5031) (-59.6275, -16.4615) (-59.5761, -16.4182) (-59.5367, -16.3818) (-59.5084, -16.3533) (-59.4901, -16.3337) (-59.4811, -16.3237) knots -1 -1 -1 -1 -1 -1 -0.98571429 -0.97142857 -0.95714286 -0.94285714 -0.92857143 -0.91428571 -0.9 -0.88571429 -0.87142857 -0.85714286 -0.84285714 -0.82857143 -0.81428571 -0.8 -0.78571429 -0.77142857 -0.75714286 -0.74285714 -0.72857143 -0.71428571 -0.7 -0.68571429 -0.67142857 -0.65714286 -0.64285714 -0.62857143 -0.61428571 -0.6 -0.58571429 -0.57142857 -0.55714286 -0.54285714 -0.52857143 -0.51428571 -0.5 -0.48571429 -0.47142857 -0.45714286 -0.44285714 -0.42857143 -0.41428571 -0.4 -0.38571429 -0.37142857 -0.35714286 -0.34285714 -0.32857143 -0.31428571 -0.3 -0.28571429 -0.27142857 -0.25714286 -0.24285714 -0.22857143 -0.21428571 -0.2 -0.18571429 -0.17142857 -0.15714286 -0.14285714 -0.12857143 -0.11428571 -0.1 -0.08571429 -0.07142857 -0.05714286 -0.04285714 -0.02857143 -0.01428571 0 0 0 0 0 0
  line L11 (-59.4811, -16.3237) -> (-58.8114, -15.585)
  arc A17 (-56.6667, -15.3936) -> (-58.8114, -15.585) centre (-57.6353, -16.6513) ccw
  arc A18 (-56.6667, -15.3936) -> (-56.0616, -15.8401) centre (-45.4614, -0.8441) ccw
  arc A19 (-55.6124, -17.946) -> (-56.0616, -15.8401) centre (-56.9779, -17.1365) ccw
  line L12 (-55.6124, -17.946) -> (-56.1208, -18.8037)
  spline S10 degree 5 poles (-56.1208, -18.8037) (-56.1277, -18.8152) (-56.141, -18.8385) (-56.1599, -18.874) (-56.1831, -18.9223) (-56.2093, -18.9842) (-56.2335, -19.047) (-56.2565, -19.1106) (-56.2788, -19.1744) (-56.3006, -19.2386) (-56.322, -19.3029) (-56.3426, -19.3676) (-56.3624, -19.4327) (-56.3813, -19.4983) (-56.3991, -19.5643) (-56.4159, -19.6308) (-56.432, -19.6976) (-56.4474, -19.7647) (-56.4622, -19.8321) (-56.4765, -19.8997) (-56.4902, -19.9675) (-56.5032, -20.0356) (-56.5157, -20.104) (-56.5275, -20.1726) (-56.5386, -20.2414) (-56.5492, -20.3105) (-56.5591, -20.3799) (-56.5685, -20.4494) (-56.5774, -20.5191) (-56.5857, -20.5891) (-56.5935, -20.6592) (-56.6007, -20.7295) (-56.6074, -20.8) (-56.6136, -20.8707) (-56.6192, -20.9416) (-56.6243, -21.0126) (-56.629, -21.0838) (-56.6331, -21.1551) (-56.6367, -21.2267) (-56.6398, -21.2983) (-56.6424, -21.3701) (-56.6446, -21.4421) (-56.6462, -21.5142) (-56.6474, -21.5864) (-56.6481, -21.6588) (-56.6483, -21.7313) (-56.648, -21.804) (-56.6473, -21.8767) (-56.6461, -21.9496) (-56.6445, -22.0226) (-56.6424, -22.0957) (-56.6398, -22.1689) (-56.6368, -22.2422) (-56.6333, -22.3157) (-56.6294, -22.3892) (-56.6251, -22.4628) (-56.6203, -22.5366) (-56.615, -22.6104) (-56.6093, -22.6843) (-56.6032, -22.7583) (-56.5967, -22.8324) (-56.5897, -22.9066) (-56.5823, -22.9809) (-56.5744, -23.0552) (-56.5662, -23.1296) (-56.5575, -23.2041) (-56.5483, -23.2787) (-56.5388, -23.3533) (-56.5288, -23.428) (-56.5184, -23.5028) (-56.5076, -23.5776) (-56.4987, -23.6375) (-56.4918, -23.6825) (-56.4871, -23.7125) (-56.4847, -23.7275) knots 0 0 0 0 0 0 0.01428571 0.02857143 0.04285714 0.05714286 0.07142857 0.08571429 0.1 0.11428571 0.12857143 0.14285714 0.15714286 0.17142857 0.18571429 0.2 0.21428571 0.22857143 0.24285714 0.25714286 0.27142857 0.28571429 0.3 0.31428571 0.32857143 0.34285714 0.35714286 0.37142857 0.38571429 0.4 0.41428571 0.42857143 0.44285714 0.45714286 0.47142857 0.48571429 0.5 0.51428571 0.52857143 0.54285714 0.55714286 0.57142857 0.58571429 0.6 0.61428571 0.62857143 0.64285714 0.65714286 0.67142857 0.68571429 0.7 0.71428571 0.72857143 0.74285714 0.75714286 0.77142857 0.78571429 0.8 0.81428571 0.82857143 0.84285714 0.85714286 0.87142857 0.88571429 0.9 0.91428571 0.92857143 0.94285714 0.95714286 0.97142857 0.98571429 1 1 1 1 1 1
  arc A20 (-56.4847, -23.7275) -> (-54.7383, -24.4894) centre (-45.4614, -0.8441) ccw
  spline S11 degree 5 poles (-54.7383, -24.4894) (-54.7257, -24.481) (-54.7005, -24.464) (-54.6628, -24.4385) (-54.6128, -24.4043) (-54.5506, -24.3613) (-54.4888, -24.3181) (-54.4272, -24.2746) (-54.366, -24.2308) (-54.3052, -24.1868) (-54.2446, -24.1425) (-54.1845, -24.098) (-54.1246, -24.0531) (-54.0651, -24.0081) (-54.006, -23.9627) (-53.9472, -23.9171) (-53.8888, -23.8713) (-53.8308, -23.8252) (-53.7731, -23.7788) (-53.7158, -23.7322) (-53.6588, -23.6853) (-53.6023, -23.6381) (-53.5461, -23.5907) (-53.4903, -23.543) (-53.4349, -23.4951) (-53.3798, -23.4469) (-53.3252, -23.3985) (-53.271, -23.3498) (-53.2171, -23.3008) (-53.1637, -23.2516) (-53.1107, -23.2021) (-53.0581, -23.1524) (-53.006, -23.1024) (-52.9543, -23.0522) (-52.903, -23.0017) (-52.8521, -22.9509) (-52.8017, -22.8999) (-52.7517, -22.8486) (-52.7022, -22.797) (-52.6531, -22.7452) (-52.6046, -22.6931) (-52.5565, -22.6408) (-52.5088, -22.5882) (-52.4617, -22.5353) (-52.4151, -22.4822) (-52.369, -22.4288) (-52.3234, -22.3751) (-52.2783, -22.3212) (-52.2337, -22.267) (-52.1896, -22.2126) (-52.1461, -22.1579) (-52.1033, -22.1028) (-52.061, -22.0475) (-52.0194, -21.9919) (-51.9783, -21.936) (-51.9379, -21.8799) (-51.8981, -21.8234) (-51.8587, -21.7667) (-51.82, -21.7098) (-51.782, -21.6526) (-51.7447, -21.595) (-51.7084, -21.537) (-51.6732, -21.4786) (-51.6389, -21.4198) (-51.6056, -21.3607) (-51.5729, -21.3012) (-51.5407, -21.2416) (-51.5091, -21.1818) (-51.4781, -21.1218) (-51.4485, -21.0613) (-51.421, -21) (-51.4013, -20.9502) (-51.3882, -20.9122) (-51.3802, -20.8866) (-51.3764, -20.8737) knots -1 -1 -1 -1 -1 -1 -0.98571429 -0.97142857 -0.95714286 -0.94285714 -0.92857143 -0.91428571 -0.9 -0.88571429 -0.87142857 -0.85714286 -0.84285714 -0.82857143 -0.81428571 -0.8 -0.78571429 -0.77142857 -0.75714286 -0.74285714 -0.72857143 -0.71428571 -0.7 -0.68571429 -0.67142857 -0.65714286 -0.64285714 -0.62857143 -0.61428571 -0.6 -0.58571429 -0.57142857 -0.55714286 -0.54285714 -0.52857143 -0.51428571 -0.5 -0.48571429 -0.47142857 -0.45714286 -0.44285714 -0.42857143 -0.41428571 -0.4 -0.38571429 -0.37142857 -0.35714286 -0.34285714 -0.32857143 -0.31428571 -0.3 -0.28571429 -0.27142857 -0.25714286 -0.24285714 -0.22857143 -0.21428571 -0.2 -0.18571429 -0.17142857 -0.15714286 -0.14285714 -0.12857143 -0.11428571 -0.1 -0.08571429 -0.07142857 -0.05714286 -0.04285714 -0.02857143 -0.01428571 0 0 0 0 0 0
  line L13 (-51.3764, -20.8737) -> (-51.0935, -19.9176)
  arc A21 (-49.2442, -18.8145) -> (-51.0935, -19.9176) centre (-49.5712, -20.368) ccw
  arc A22 (-49.2442, -18.8145) -> (-48.5053, -18.9543) centre (-45.4614, -0.8441) ccw
  arc A23 (-47.1869, -20.6568) -> (-48.5053, -18.9543) centre (-48.7685, -20.5199) ccw
  line L14 (-47.1869, -20.6568) -> (-47.2729, -21.6501)
  spline S12 degree 5 poles (-47.2729, -21.6501) (-47.274, -21.6635) (-47.2759, -21.6902) (-47.2776, -21.7304) (-47.2775, -21.784) (-47.2743, -21.8511) (-47.2688, -21.9182) (-47.2619, -21.9854) (-47.2543, -22.0527) (-47.2461, -22.1199) (-47.2375, -22.1872) (-47.228, -22.2544) (-47.2176, -22.3217) (-47.2061, -22.3889) (-47.1935, -22.4561) (-47.1799, -22.5233) (-47.1654, -22.5905) (-47.1501, -22.6577) (-47.1342, -22.7248) (-47.1177, -22.7919) (-47.1006, -22.8589) (-47.0829, -22.9259) (-47.0644, -22.9929) (-47.0453, -23.0599) (-47.0255, -23.1267) (-47.005, -23.1936) (-46.9839, -23.2604) (-46.9622, -23.3271) (-46.9399, -23.3938) (-46.917, -23.4604) (-46.8936, -23.5269) (-46.8696, -23.5934) (-46.8451, -23.6598) (-46.82, -23.7262) (-46.7943, -23.7925) (-46.7681, -23.8587) (-46.7414, -23.9249) (-46.7141, -23.9909) (-46.6863, -24.0569) (-46.658, -24.1229) (-46.6292, -24.1887) (-46.5999, -24.2545) (-46.5702, -24.3201) (-46.5399, -24.3857) (-46.5091, -24.4512) (-46.4778, -24.5167) (-46.4461, -24.582) (-46.4139, -24.6472) (-46.3812, -24.7124) (-46.348, -24.7774) (-46.3144, -24.8424) (-46.2803, -24.9072) (-46.2458, -24.972) (-46.2108, -25.0367) (-46.1754, -25.1012) (-46.1395, -25.1657) (-46.1032, -25.23) (-46.0664, -25.2943) (-46.0292, -25.3584) (-45.9916, -25.4224) (-45.9536, -25.4863) (-45.9151, -25.5501) (-45.8762, -25.6138) (-45.8369, -25.6774) (-45.7971, -25.7409) (-45.757, -25.8042) (-45.7164, -25.8674) (-45.6754, -25.9305) (-45.634, -25.9935) (-45.5922, -26.0564) (-45.55, -26.1191) (-45.516, -26.1692) (-45.4902, -26.2067) (-45.473, -26.2317) (-45.4643, -26.2441) knots 0 0 0 0 0 0 0.01428571 0.02857143 0.04285714 0.05714286 0.07142857 0.08571429 0.1 0.11428571 0.12857143 0.14285714 0.15714286 0.17142857 0.18571429 0.2 0.21428571 0.22857143 0.24285714 0.25714286 0.27142857 0.28571429 0.3 0.31428571 0.32857143 0.34285714 0.35714286 0.37142857 0.38571429 0.4 0.41428571 0.42857143 0.44285714 0.45714286 0.47142857 0.48571429 0.5 0.51428571 0.52857143 0.54285714 0.55714286 0.57142857 0.58571429 0.6 0.61428571 0.62857143 0.64285714 0.65714286 0.67142857 0.68571429 0.7 0.71428571 0.72857143 0.74285714 0.75714286 0.77142857 0.78571429 0.8 0.81428571 0.82857143 0.84285714 0.85714286 0.87142857 0.88571429 0.9 0.91428571 0.92857143 0.94285714 0.95714286 0.97142857 0.98571429 1 1 1 1 1 1
  arc A24 (-45.4643, -26.2441) -> (-43.5603, -26.1729) centre (-45.4614, -0.8441) ccw
  spline S13 degree 5 poles (-43.5603, -26.1729) (-43.5526, -26.1598) (-43.5373, -26.1336) (-43.5144, -26.0943) (-43.4842, -26.0418) (-43.4468, -25.9761) (-43.4098, -25.9103) (-43.3732, -25.8444) (-43.3371, -25.7784) (-43.3013, -25.7123) (-43.266, -25.6462) (-43.2311, -25.5799) (-43.1967, -25.5136) (-43.1626, -25.4471) (-43.129, -25.3806) (-43.0959, -25.3141) (-43.0631, -25.2474) (-43.0308, -25.1807) (-42.999, -25.1139) (-42.9676, -25.047) (-42.9366, -24.98) (-42.9061, -24.913) (-42.8761, -24.8459) (-42.8465, -24.7788) (-42.8173, -24.7115) (-42.7887, -24.6442) (-42.7605, -24.5769) (-42.7327, -24.5095) (-42.7055, -24.442) (-42.6787, -24.3745) (-42.6524, -24.3069) (-42.6266, -24.2393) (-42.6013, -24.1716) (-42.5765, -24.1039) (-42.5522, -24.0362) (-42.5284, -23.9683) (-42.5052, -23.9005) (-42.4824, -23.8326) (-42.4601, -23.7647) (-42.4384, -23.6967) (-42.4172, -23.6287) (-42.3966, -23.5607) (-42.3765, -23.4926) (-42.357, -23.4246) (-42.3381, -23.3565) (-42.3197, -23.2884) (-42.3019, -23.2202) (-42.2846, -23.1521) (-42.268, -23.0839) (-42.2519, -23.0157) (-42.2365, -22.9475) (-42.2217, -22.8794) (-42.2076, -22.8112) (-42.1942, -22.743) (-42.1815, -22.6749) (-42.1695, -22.6067) (-42.1581, -22.5386) (-42.1472, -22.4705) (-42.137, -22.4024) (-42.1276, -22.3343) (-42.119, -22.2663) (-42.1115, -22.1983) (-42.105, -22.1304) (-42.0997, -22.0625) (-42.0953, -21.9948) (-42.0917, -21.927) (-42.0886, -21.8594) (-42.086, -21.7918) (-42.0841, -21.7242) (-42.0837, -21.6569) (-42.0855, -21.5897) (-42.0894, -21.5363) (-42.0941, -21.4963) (-42.098, -21.4698) (-42.1001, -21.4566) knots -1 -1 -1 -1 -1 -1 -0.98571429 -0.97142857 -0.95714286 -0.94285714 -0.92857143 -0.91428571 -0.9 -0.88571429 -0.87142857 -0.85714286 -0.84285714 -0.82857143 -0.81428571 -0.8 -0.78571429 -0.77142857 -0.75714286 -0.74285714 -0.72857143 -0.71428571 -0.7 -0.68571429 -0.67142857 -0.65714286 -0.64285714 -0.62857143 -0.61428571 -0.6 -0.58571429 -0.57142857 -0.55714286 -0.54285714 -0.52857143 -0.51428571 -0.5 -0.48571429 -0.47142857 -0.45714286 -0.44285714 -0.42857143 -0.41428571 -0.4 -0.38571429 -0.37142857 -0.35714286 -0.34285714 -0.32857143 -0.31428571 -0.3 -0.28571429 -0.27142857 -0.25714286 -0.24285714 -0.22857143 -0.21428571 -0.2 -0.18571429 -0.17142857 -0.15714286 -0.14285714 -0.12857143 -0.11428571 -0.1 -0.08571429 -0.07142857 -0.05714286 -0.04285714 -0.02857143 -0.01428571 0 0 0 0 0 0
  line L15 (-42.1001, -21.4566) -> (-42.2601, -20.4724)
  arc A25 (-41.0726, -18.6762) -> (-42.2601, -20.4724) centre (-40.6932, -20.2177) ccw
  arc A26 (-41.0726, -18.6762) -> (-40.3462, -18.4816) centre (-45.4614, -0.8441) ccw
  arc A27 (-38.4196, -19.4434) -> (-40.3462, -18.4816) centre (-39.904, -20.0062) ccw
  line L16 (-38.4196, -19.4434) -> (-38.0661, -20.3756)
  spline S14 degree 5 poles (-38.0661, -20.3756) (-38.0613, -20.3882) (-38.0515, -20.4131) (-38.0355, -20.45) (-38.0122, -20.4983) (-37.9802, -20.5573) (-37.9461, -20.6155) (-37.9108, -20.673) (-37.8747, -20.7303) (-37.8382, -20.7873) (-37.8012, -20.8441) (-37.7635, -20.9006) (-37.725, -20.9567) (-37.6854, -21.0123) (-37.6449, -21.0674) (-37.6034, -21.122) (-37.5612, -21.1763) (-37.5183, -21.2302) (-37.4749, -21.2837) (-37.4309, -21.337) (-37.3864, -21.39) (-37.3414, -21.4427) (-37.2957, -21.495) (-37.2494, -21.547) (-37.2025, -21.5987) (-37.1551, -21.65) (-37.1071, -21.701) (-37.0586, -21.7517) (-37.0095, -21.8021) (-36.96, -21.8522) (-36.9101, -21.902) (-36.8596, -21.9515) (-36.8087, -22.0007) (-36.7573, -22.0496) (-36.7054, -22.0982) (-36.653, -22.1465) (-36.6003, -22.1945) (-36.547, -22.2422) (-36.4934, -22.2896) (-36.4393, -22.3368) (-36.3848, -22.3836) (-36.3298, -22.4301) (-36.2745, -22.4764) (-36.2187, -22.5223) (-36.1626, -22.568) (-36.106, -22.6134) (-36.0491, -22.6585) (-35.9918, -22.7033) (-35.9341, -22.7478) (-35.876, -22.792) (-35.8175, -22.8359) (-35.7586, -22.8796) (-35.6994, -22.9229) (-35.6399, -22.966) (-35.5799, -23.0088) (-35.5196, -23.0513) (-35.459, -23.0935) (-35.398, -23.1355) (-35.3367, -23.1771) (-35.275, -23.2185) (-35.213, -23.2595) (-35.1506, -23.3003) (-35.0879, -23.3408) (-35.0249, -23.3811) (-34.9616, -23.421) (-34.8979, -23.4606) (-34.8339, -23.5) (-34.7696, -23.5391) (-34.705, -23.5778) (-34.6401, -23.6163) (-34.5749, -23.6545) (-34.5224, -23.6849) (-34.483, -23.7075) (-34.4566, -23.7225) (-34.4434, -23.73) knots 0 0 0 0 0 0 0.01428571 0.02857143 0.04285714 0.05714286 0.07142857 0.08571429 0.1 0.11428571 0.12857143 0.14285714 0.15714286 0.17142857 0.18571429 0.2 0.21428571 0.22857143 0.24285714 0.25714286 0.27142857 0.28571429 0.3 0.31428571 0.32857143 0.34285714 0.35714286 0.37142857 0.38571429 0.4 0.41428571 0.42857143 0.44285714 0.45714286 0.47142857 0.48571429 0.5 0.51428571 0.52857143 0.54285714 0.55714286 0.57142857 0.58571429 0.6 0.61428571 0.62857143 0.64285714 0.65714286 0.67142857 0.68571429 0.7 0.71428571 0.72857143 0.74285714 0.75714286 0.77142857 0.78571429 0.8 0.81428571 0.82857143 0.84285714 0.85714286 0.87142857 0.88571429 0.9 0.91428571 0.92857143 0.94285714 0.95714286 0.97142857 0.98571429 1 1 1 1 1 1
  arc A28 (-34.4434, -23.73) -> (-32.7588, -22.8397) centre (-45.4614, -0.8441) ccw
  spline S15 degree 5 poles (-32.7588, -22.8397) (-32.7576, -22.8246) (-32.7551, -22.7943) (-32.7516, -22.749) (-32.7471, -22.6886) (-32.7419, -22.6131) (-32.7372, -22.5378) (-32.7328, -22.4626) (-32.7289, -22.3874) (-32.7254, -22.3124) (-32.7223, -22.2375) (-32.7196, -22.1626) (-32.7173, -22.0879) (-32.7154, -22.0133) (-32.714, -21.9388) (-32.713, -21.8644) (-32.7125, -21.7902) (-32.7123, -21.716) (-32.7126, -21.642) (-32.7133, -21.5681) (-32.7145, -21.4944) (-32.7161, -21.4208) (-32.7181, -21.3473) (-32.7206, -21.2739) (-32.7235, -21.2007) (-32.7269, -21.1277) (-32.7307, -21.0547) (-32.735, -20.982) (-32.7397, -20.9094) (-32.7448, -20.8369) (-32.7505, -20.7646) (-32.7566, -20.6925) (-32.7631, -20.6206) (-32.7702, -20.5488) (-32.7777, -20.4772) (-32.7857, -20.4058) (-32.7941, -20.3345) (-32.8031, -20.2635) (-32.8125, -20.1926) (-32.8224, -20.122) (-32.8328, -20.0515) (-32.8438, -19.9813) (-32.8552, -19.9113) (-32.8672, -19.8415) (-32.8796, -19.7719) (-32.8926, -19.7026) (-32.9062, -19.6334) (-32.9202, -19.5646) (-32.9347, -19.4959) (-32.9499, -19.4275) (-32.9655, -19.3594) (-32.9818, -19.2916) (-32.9987, -19.224) (-33.0162, -19.1568) (-33.0343, -19.0899) (-33.0531, -19.0233) (-33.0723, -18.9569) (-33.0921, -18.8908) (-33.1125, -18.8251) (-33.1335, -18.7596) (-33.1553, -18.6946) (-33.178, -18.6301) (-33.2017, -18.5661) (-33.2263, -18.5027) (-33.2517, -18.4397) (-33.2778, -18.3771) (-33.3044, -18.3148) (-33.3314, -18.2528) (-33.3591, -18.1911) (-33.3879, -18.1302) (-33.4186, -18.0705) (-33.4453, -18.0241) (-33.4669, -17.9901) (-33.4819, -17.9679) (-33.4896, -17.9569) knots -1 -1 -1 -1 -1 -1 -0.98571429 -0.97142857 -0.95714286 -0.94285714 -0.92857143 -0.91428571 -0.9 -0.88571429 -0.87142857 -0.85714286 -0.84285714 -0.82857143 -0.81428571 -0.8 -0.78571429 -0.77142857 -0.75714286 -0.74285714 -0.72857143 -0.71428571 -0.7 -0.68571429 -0.67142857 -0.65714286 -0.64285714 -0.62857143 -0.61428571 -0.6 -0.58571429 -0.57142857 -0.55714286 -0.54285714 -0.52857143 -0.51428571 -0.5 -0.48571429 -0.47142857 -0.45714286 -0.44285714 -0.42857143 -0.41428571 -0.4 -0.38571429 -0.37142857 -0.35714286 -0.34285714 -0.32857143 -0.31428571 -0.3 -0.28571429 -0.27142857 -0.25714286 -0.24285714 -0.22857143 -0.21428571 -0.2 -0.18571429 -0.17142857 -0.15714286 -0.14285714 -0.12857143 -0.11428571 -0.1 -0.08571429 -0.07142857 -0.05714286 -0.04285714 -0.02857143 -0.01428571 0 0 0 0 0 0
  line L17 (-33.4896, -17.9569) -> (-34.0607, -17.1396)
  arc A29 (-33.7702, -15.006) -> (-34.0607, -17.1396) centre (-32.7595, -16.2303) ccw
  arc A30 (-33.7702, -15.006) -> (-33.2001, -14.5155) centre (-45.4614, -0.8441) ccw
  arc A31 (-31.0471, -14.5462) -> (-33.2001, -14.5155) centre (-32.1402, -15.6973) ccw
  line L18 (-31.0471, -14.5462) -> (-30.3241, -15.2327)